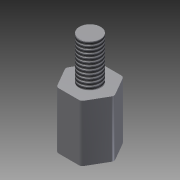
# Autodesk Inventor part: Spacer(M3-8mm)
Saved by Autodesk Inventor 2012 (Build 160160000, 160)
## iProperties
Created: 2013-02-09
Material: Default
Document SubType Name: Modeling
Designer: andou
Density: 1 g/cm^3
Author: andou
Title: Spacer(M3-8mm)
Autodesk Inventor part; units mm, degrees
ref_plane "YZ Plane" through (0, 0, 0) normal (1, 0, 0) x (0, 1, 0)
ref_plane "XZ Plane" through (0, 0, 0) normal (0, 1, 0) x (-1, 0, 0)
ref_plane "XY Plane" through (0, 0, 0) normal (0, 0, 1) x (1, 0, 0)
sketch "スケッチ1" plane through (0, 0, 0) normal (0, 0, 1) x (1, 0, 0)
  line L0 (1.7321, -3) -> (-1.7321, -3)
  line L1 (-1.7321, -3) -> (-3.4641, 0)
  line L2 (-3.4641, 0) -> (-1.7321, 3)
  line L3 (-1.7321, 3) -> (1.7321, 3)
  line L4 (1.7321, 3) -> (3.4641, 0)
  line L5 (3.4641, 0) -> (1.7321, -3)
  point P0 (0, 0)
  point P1 (0, 0)
  dimension "d5" = 6
  dimension "d6" = 3
  constraints: 12 end point, 13 other
  measures "d5" distance between parallel lines of L0 L3
  measures "d6" vertical distance of L3.end L4.end
extrude "押し出し1" add sketch "スケッチ1" along normal blind 8
sketch "スケッチ2" plane through (0, 0, 8) normal (0, 0, 1) x (1, 0, 0)
  circle A0 centre (0, 0) radius 1.5
  dimension "d10" = 3
  constraints: 1 centre point, 1 coincident
  measures "d10" diameter of A0
extrude "押し出し2" add sketch "スケッチ2" along normal blind 6
sketch "スケッチ3" plane through (0, 0, 0) normal (0, 0, -1) x (-1, 0, 0)
  circle A0 centre (0, 0) radius 1.5
  dimension "d13" = 3
  constraints: 1 centre point, 1 coincident
  measures "d13" diameter of A0
hole "穴1" at (0, 0, 0) direction (0, 0, 1) diameter 3 depth 6 tip angle 118
thread "ねじ1" size "M3x0.5" class "6g" standard "ANSI Metric M Profile" full length
thread "ねじ2" size "M3x0.5" class "6H" standard "ANSI Metric M Profile" full length
fillet "フィレット1" radius 0.5 6 edges at (-3.4641, 0, 4) (-1.7321, -3, 4) (-1.7321, 3, 4) (1.7321, 3, 4) (3.4641, 0, 4) (1.7321, -3, 4)
